littleproximalphalanx (Autodesk Fusion 360 design; units mm, degrees)
Autodesk Fusion 360 part; units mm, degrees
sketch "Sketch1" plane through (0, 0, 0) normal (0, 0, 1) x (1, 0, 0)
  line L0 (10, 5) -> (-10, 5)
  line L1 (-10, 5) -> (-10, -5)
  line L2 (-10, -5) -> (10, -5)
  line L3 (10, -5) -> (10, 5)
  line L4 (10, 5) -> (-10, -5) construction
  line L5 (-10, 5) -> (10, -5) construction
  circle A0 centre (10, 0) radius 5
  circle A1 centre (-17.5, 0) radius 10
  circle A2 centre (11.6583, 2.5) radius 0.75
  line L6 (-10, 5) -> (10, 5)
  line L7 (10, 5) -> (10, 6)
  line L8 (10, 6) -> (-10, 6)
  line L9 (-10, 6) -> (-10, 5)
  circle A3 centre (-17.5, 0) radius 5
  line L10 (5, 0) -> (5, 5)
  line L11 (5, 0) -> (5, -5)
  circle A4 centre (10, 0) radius 0.85
  line L12 (-4.5, -1.75) -> (0.5, -1.75)
  arc A5 (0.5, -1.75) -> (0.5, 1.75) centre (0.5, 0) ccw
  line L13 (0.5, 1.75) -> (-4.5, 1.75)
  arc A6 (-4.5, 1.75) -> (-4.5, -1.75) centre (-4.5, 0) ccw
  line L14 (-4.5, 0) -> (0.5, 0) construction
  circle A7 centre (11.6583, 2.5) radius 1.5
  spline S0 degree 5 poles (11.265, 4.8373) (11.146, 4.8061) (10.9173, 4.7371) (10.6018, 4.6143) (10.2365, 4.412) (9.8725, 4.0955) (9.5992, 3.7201) (9.4117, 3.2965) (9.2992, 2.8441) (9.2446, 2.3917) (9.2262, 1.9617) (9.2204, 1.5581) (9.2027, 1.1477) (9.1515, 0.6556) (9.0567, 0.0734) (8.9151, -0.581) (8.7287, -1.2661) (8.5022, -1.9336) (8.2409, -2.539) (7.9486, -3.0546) (7.6278, -3.4653) (7.3497, -3.7046) (7.1294, -3.8334) (6.9773, -3.8969) (6.9, -3.923) knots 0 0 0 0 0 0 0.05 0.1 0.15 0.2 0.25 0.3 0.35 0.4 0.45 0.5 0.55 0.6 0.65 0.7 0.75 0.8 0.85 0.9 0.95 1 1 1 1 1 1
  line L15 (6.9, -3.923) -> (6.9, -5)
  circle A8 centre (-17.5, 0) radius 10.5
  line L16 (9.25, 2.272) -> (9.1744, 0.5691)
  point P0 (9.4583, 3.3661)
  point P1 (9.2122, 1.4206)
  point P2 (8.5, -1.9012)
  dimension "d1" = 20
  dimension "d2" = 10
  dimension "d6" = 20
  dimension "d7" = 7.5
  dimension "d8" = 5
  dimension "d9" = 1.5
  dimension "d10" = 3
  dimension "d12" = 2.5
  dimension "d13" = 20
  dimension "d14" = 1
  dimension "d15" = 10
  dimension "d31" = 1.7
  dimension "d35" = 3.5
  dimension "d36" = 3.25
  dimension "d47" = 3
  dimension "d57" = 21
  dimension "d79" = 2.2
  dimension "d80" = 0.75
  dimension "d81" = 1.5
  dimension "d82" = 1.265
  dimension "d83" = 3.1
  dimension "d84" = 4.5
  dimension "d85" = 13
  constraint horizontal L0
  constraint perpendicular L0 L1
  constraint parallel L0 L2
  constraint parallel L1 L3
  constraint coincident L4 origin
  constraint coincident L5 origin
  constraint midpoint L3 A0.centre
  constraint coincident L2.end A0
  constraint horizontal L6
  constraint vertical L7
  constraint horizontal L8
  constraint vertical L9
  constraint concentric A1 A3
  constraint coincident A0 L10.start
  constraint coincident L0 L10.end
  constraint tangent A0 L10
  constraint perpendicular L0 L10
  constraint coincident L2 L11.end
  constraint tangent A0 L11
  constraint concentric A0 A4
  constraint tangent L12 A5
  constraint tangent A5 L13
  constraint parallel L12 L13
  constraint tangent L13 A6
  constraint tangent L12 A6
  constraint perpendicular L10 L14
  constraint concentric A2 A7
  constraint coincident A0 S0.start
  constraint coincident A0 S0.end
  constraint coincident L2 L15.end
  constraint perpendicular L2 L15
  constraint concentric A1 A8
  constraint midpoint P1 L16
  constraint tangent A4 L16
  measures "d1" distance of L1.end L2.end
  measures "d2" distance of L0.end L1.end
  measures "d6" diameter of A1
  measures "d7" distance of L1 A1.centre
  measures "d8" distance of L2 A1.centre
  measures "d9" diameter of A2
  measures "d10" distance of A0.centre A2.centre
  measures "d12" vertical distance of A0.centre A2.centre
  measures "d13" distance of L0.end L0.start
  measures "d14" distance of L0.end L8.end
  measures "d15" diameter of A3
  measures "d31" diameter of A4
  measures "d35" diameter of A5
  measures "d36" distance of L0 L13
  measures "d47" diameter of A7
  measures "d57" diameter of A8
  measures "d79" horizontal distance of A2.centre P0
  measures "d80" distance of L3 L16.start
  measures "d81" distance of L3 P2
  measures "d82" distance of L3 S0.start
  measures "d83" distance of L3 S0.end
  measures "d84" distance of L11 A5.centre
  measures "d85" distance of A1.centre A6.centre
extrude "Extrude1" add sketch "Sketch1" along normal blind 3 contours L0 A0 L6 L10 | L3 A0 S0 | L3 A0 S0 | L0 L6 L7 L8 A8 | L0 L2 L6 L10 L11 A8 | L3 A0 A4 S0 | L3 A0 A4 S0 | L2 A0 L11 L15 | L0 L2 A1 L6 A8 | L0 A1 L6 L8 A8 | L3 A4 | L3 A4 | L2 A0 L15 | L0 L1 L2 A1 L6 | L0 A1 L6 L8 L9 | L1 L2 A1 L8 L9 | A2 | L12 A5 L13 A6 | A7
extrude "Extrude2" cut sketch "Sketch1" along normal blind 1.5 contours L3 A0 S0 | L3 A0 S0 | L3 A0 A4 S0 | L3 A0 A4 S0 | L3 A4 | L3 A4 | A7
extrude "Extrude3" cut sketch "Sketch1" along normal blind 1.5 contours L2 A0 L11 L15 | L2 A0 L15
extrude "Extrude4" cut sketch "Sketch1" along normal blind 1.5 contours A2
extrude "Extrude5" add sketch "Sketch1" along normal blind 7 contours A2
extrude "Extrude6" cut sketch "Sketch1" along normal blind 1.5 contours A2
extrude "Extrude7" add sketch "Sketch1" along normal blind 1.5 contours L3 A4 | L3 A4
ref_plane "WorkPlane1" through (-6.0771, 0.2545, 5) normal (0, 0, 1) x (1, 0, 0)
mirror "Mirror1" about plane through (-6.0771, 0.2545, 5) normal (0, 0, 1) of bodies 1 merged
extrude "Extrude8" add sketch "Sketch1" along normal blind 7 contours L0 A0 L6 L10 | L0 L6 L7 L8 A8 | L0 L2 L6 L10 L11 A8 | L0 L2 A1 L6 A8 | L0 A1 L6 L8 A8
extrude "Extrude9" cut sketch "Sketch1" along normal blind 15 contours L12 A5 L13 A6
fillet "Fillet2" radius 10 4 edges at (-8.8397, -5, 8.5) (-8.8397, -5, 1.5) (-9.5, 6, 8.5) (-9.5, 6, 1.5)
extrude "Extrude10" add sketch "Sketch1" along normal blind 4 from surface at 3 contours L3 A0 S0 | L3 A0 S0 | L2 A0 L11 L15
fillet "Fillet3" radius 10 1 edges at (6.9, -3.923, 5)
fillet "Fillet5" radius 8 2 edges at (5, -5, 9.25) (5, -5, 0.75)
extrude "Extrude11" cut sketch "Sketch1" along normal blind 7 contours L0 L2 A1 L6 A8
extrude "Extrude12" add sketch "Sketch1" along normal blind 3 contours L0 L2 A1 L6 A8
extrude "Extrude13" cut sketch "Sketch1" along normal blind 7 contours L0 A1 L6 L8 L9
extrude "Extrude14" cut sketch "Sketch1" along normal blind 7 contours L0 A1 L6 L8 A8
extrude "Extrude15" add sketch "Sketch1" along normal blind 3 contours L0 A1 L6 L8 A8 | L0 A1 L6 L8 L9
fillet "Fillet8" radius 1 14 edges at (2.25, 6, 10) (-8.6623, 6.5132, 10) (-27.4922, -0.3961, 10) (-7.8068, -5.6459, 10) (-3.4602, -5, 10) (2.3123, -3.2757, 10) (6.8991, 3.9223, 10) (2.25, 6, 0) (-8.6623, 6.5132, 0) (-27.4922, -0.3961, 0) (-7.8068, -5.6459, 0) (-3.4602, -5, 0) (2.3123, -3.2757, 0) (6.8991, 3.9223, 0)
move_face "OffsetFaces1" [suppressed]
move_face "OffsetFaces2" [suppressed]
move_face "OffsetFaces3" [suppressed]
move_face "OffsetFaces4" [suppressed]
move_face "OffsetFaces5" [suppressed]
move_face "OffsetFaces6" [suppressed]
move_face "OffsetFaces7" [suppressed]
delete_face "DeleteFace1" [suppressed]
fillet "Fillet6" [suppressed]
fillet "Fillet7" [suppressed]
equation "d1 = length"
equation "d2 = thickness"
equation "length = 20 mm"
equation "thickness = 10 mm"
equation "gap = 0.3 mm"
equation "d13 = length"
equation "d31 = 2 mm - gap"
equation "d69 = -gap"
equation "d70 = -gap"
equation "d71 = -gap"
equation "d72 = -gap"
equation "d73 = -gap"
equation "d74 = -gap"
